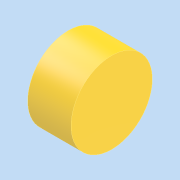
# Autodesk Inventor part: Dekel unten Plattform
Saved by Autodesk Inventor 2021 (Build 250183000, 183)
## iProperties
Created: 2024-03-14
Part Number: Dekel unten Plattform
Material: Generic
Document SubType Name: Modeling
Designer: Nokia
Density: 1 g/cm^3
Appearance: Glossy - Gold
Author: Nokia
Autodesk Inventor part; units mm, degrees
ref_plane "YZ Plane" through (0, 0, 0) normal (1, 0, 0) x (0, 1, 0)
ref_plane "XZ Plane" through (0, 0, 0) normal (0, 1, 0) x (-1, 0, 0)
ref_plane "XY Plane" through (0, 0, 0) normal (0, 0, 1) x (1, 0, 0)
sketch "Sketch1" plane through (0, 0, 0) normal (0, 0, 1) x (1, 0, 0)
  line L0 (1.5, -8.5) -> (-6.9947, -8.5)
  line L1 (1.5, -8.5) -> (1.5, 21.5)
  line L2 (1.5, 21.5) -> (-30.5, 21.5)
  line L3 (-30.5, 21.5) -> (-30.5, 19.5)
  line L4 (-30.5, 19.5) -> (-0.5, 19.5)
  line L5 (-0.5, 19.5) -> (-0.5, -8.5)
  point P0 (0, 0)
  dimension "d0" = 30
  dimension "d1" = 32
  dimension "d2" = 2
  dimension "d3" = 30
  constraints: 12 end point, 4 perpendicular, 1 horizontal, 1 point on line, 1 vertical
  measures "d0" distance of L0.start L1.end
  measures "d1" distance of L1.end L2.end
  measures "d2" distance of L2.end L3.end
  measures "d3" distance of L3.end L4.end
revolve "Revolution1" add sketch "Sketch1" angle 360 about axis through (1.5, -8.5, 0) along (-1, 0, 0)
body "Solid1"
